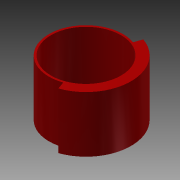
# Autodesk Inventor part: PG35LHeatSink
Saved by Autodesk Inventor 2015 (Build 190159000, 159)
## iProperties
Created: 2014-06-19
Part Number: PG35LHeatSink
Material: Generic
Document SubType Name: Modeling
Designer: Jack
Density: 1 g/cm^3
Appearance: Smooth - Red
Author: Jack
Autodesk Inventor part; units mm, degrees
ref_plane "YZ Plane" through (0, 0, 0) normal (1, 0, 0) x (0, 1, 0)
ref_plane "XZ Plane" through (0, 0, 0) normal (0, 1, 0) x (-1, 0, 0)
ref_plane "XY Plane" through (0, 0, 0) normal (0, 0, 1) x (1, 0, 0)
sketch "Sketch1" plane through (0, 0, 0) normal (0, 0, 1) x (1, 0, 0)
  circle A0 centre (0, 0) radius 17.5
  arc A1 (7.4068, -21.2459) -> (7.4068, 21.2459) centre (0, 0) ccw
  arc A2 (6.0901, 17.4689) -> (6.0901, -17.4689) centre (0, 0) ccw
  line L0 (5.7609, 21.75) -> (5.7609, 16.5246) construction
  line L1 (5.7609, -16.5246) -> (5.7609, -21.75) construction
  line L2 (6.0901, -17.4689) -> (7.4068, -21.2459)
  line L3 (6.0901, 17.4689) -> (7.4068, 21.2459)
  dimension "d0" = 35
  dimension "d1" = 45
  dimension "d2" = 43.5
  dimension "d3" = 37
  dimension "d4" = 1.646
  dimension "d5" = 0.5041
  dimension "d6" = 1.646
  dimension "d7" = 0.5041
  constraints: 8 end point, 6 point on circle, 3 centre point, 3 coincident, 2 point on line, 2 vertical, 1 vertical alignment
  measures "d0" diameter of A0
  measures "d1" diameter of A1
  measures "d2" distance of L0.start L1.end
  measures "d3" diameter of A2
  measures "d4" horizontal distance of L1.end L2.end
  measures "d5" vertical distance of L2.end L1.end
  measures "d6" horizontal distance of L3.end L0.start
  measures "d7" vertical distance of L3.end L0.start
extrude "Extrusion1" add sketch "Sketch1" along normal blind 28
body "Solid1"
